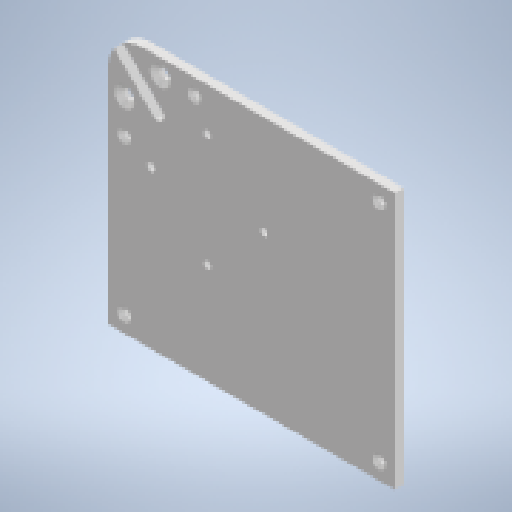
# Autodesk Inventor part: Mount plate UR
Saved by Autodesk Inventor 2024 (Build 280153000, 153)
## iProperties
Created: 2024-03-26
Part Number: Mount plate UR
Material: Generic
Document SubType Name: Modeling
Designer: jens1
Density: 1 g/cm^3
Appearance: Default
Author: jens1
Autodesk Inventor part; units mm, degrees
ref_plane "YZ Plane" through (0, 0, 0) normal (1, 0, 0) x (0, 1, 0)
ref_plane "XZ Plane" through (0, 0, 0) normal (0, 1, 0) x (-1, 0, 0)
ref_plane "XY Plane" through (0, 0, 0) normal (0, 0, 1) x (1, 0, 0)
sketch "Sketch1" plane through (0, 0, 0) normal (0, 0, 1) x (1, 0, 0)
  line L0 (0, 0) -> (335, 0)
  line L1 (335, 0) -> (335, 300)
  line L2 (335, 300) -> (0, 300)
  line L3 (0, 300) -> (0, 0)
  dimension "d0" = 335
  dimension "d1" = 300
  constraints: 8 end point, 2 parallel, 1 horizontal, 1 perpendicular
  measures "d0" distance of L2.end L1.end
  measures "d1" distance of L1.end L0.end
extrude "Plate" add sketch "Sketch1" along normal blind 10.5
sketch "Sketch3" plane through (0, 0, 10.5) normal (0, 0, 1) x (1, 0, 0)
  circle A0 centre (316.15, 18.85) radius 7.85
  line L0 (335, 0) -> (335, 300) projected
  line L1 (0, 0) -> (335, 0) projected
  circle A1 centre (316.15, 18.85) radius 4
  line L2 (0, 300) -> (0, 0) projected
  line L3 (335, 300) -> (0, 300) projected
  circle A2 centre (18.85, 199.55) radius 7.85
  circle A3 centre (100.45, 281.15) radius 7.85
  point P0 (18.85, 18.85)
  point P1 (316.15, 281.15)
  dimension "d4" = 15.7
  dimension "d5" = 18.85
  dimension "d6" = 18.85
  dimension "d7" = 8
  dimension "d8" = 18.85
  dimension "d9" = 18.85
  dimension "d10" = 18.85
  dimension "d11" = 18.85
  dimension "d19" = 18.85
  dimension "d20" = 18.85
  dimension "d21" = 15.7
  dimension "d22" = 15.7
  dimension "d23" = 180.7
  dimension "d24" = 215.7
  constraints: 4 centre point, 3 coincident
  measures "d4" diameter of A0
  measures "d5" distance from line of L0 A0.centre
  measures "d6" distance from line of L1 A0.centre
  measures "d7" diameter of A1
  measures "d8" distance from line of point (18.85, 18.85) L1
  measures "d9" distance from line of L2 point (18.85, 18.85)
  measures "d10" distance from line of L0 point (316.15, 281.15)
  measures "d11" distance from line of L3 point (316.15, 281.15)
  measures "d19" distance from line of L3 point (100.45, 281.15)
  measures "d20" distance from line of L2 point (18.85, 199.55)
  measures "d21" diameter of A3
  measures "d22" diameter of A2
  measures "d23" distance of point (18.85, 18.85) A2.centre
  measures "d24" distance of point (316.15, 281.15) point (100.45, 281.15)
hole "Small screw" at (18.85, 18.85, 10.5) at (316.15, 281.15, 10.5) at (316.15, 18.85, 10.5) at (18.85, 199.55, 10.5) at (100.45, 281.15, 10.5) direction (0, 0, -1) diameter 8 end through all countersink diameter 15.7 countersink angle 90
sketch "Sketch4" plane through (0, 0, 10.5) normal (0, 0, 1) x (1, 0, 0)
  circle A0 centre (100.45, 281.15) radius 7.85 projected
  circle A1 centre (18.85, 199.55) radius 7.85 projected
  circle A2 centre (18.85, 239.15) radius 11.75
  circle A3 centre (60.85, 281.15) radius 11.75
  circle A4 centre (18.85, 199.55) radius 4 projected
  circle A5 centre (18.85, 199.55) radius 7.85
  point P0 (0, 0)
  dimension "d25" = 23.5
  dimension "d26" = 23.5
  dimension "d27" = 0
  dimension "d28" = 0
  dimension "d29" = 39.6
  dimension "d30" = 15.7
  dimension "d31" = 39.6
  constraints: 3 centre point, 3 coincident
  measures "d25" diameter of A2
  measures "d26" diameter of A3
  measures "d27" vertical distance of A0.centre point (60.85, 281.15)
  measures "d28" horizontal distance of A1.centre point (18.85, 239.15)
  measures "d29" distance of point (18.85, 239.15) A1.centre
  measures "d30" diameter of A5
  measures "d31" distance of A0.centre A3.centre
hole "Big screw" at (60.85, 281.15, 10.5) at (18.85, 239.15, 10.5) direction (0, 0, -1) diameter 12 end through all countersink diameter 23.5 countersink angle 90
fillet "Stor runding" radius 40 1 edges at (0, 300, 5.25)
sketch "Sketch6" plane through (0, 0, 10.5) normal (0, 0, 1) x (1, 0, 0)
  arc A0 (40, 300) -> (0, 260) centre (40, 260) ccw projected
  line L0 (0, 260) -> (0, 0) projected
  line L1 (0, 0) -> (335, 0) projected
  line L2 (335, 0) -> (335, 300) projected
  line L3 (335, 300) -> (40, 300) projected
  circle A1 centre (18.85, 239.15) radius 11.75 projected
  circle A2 centre (60.85, 281.15) radius 11.75 projected
  circle A3 centre (100.45, 281.15) radius 7.85 projected
  circle A4 centre (18.85, 199.55) radius 7.85 projected
  circle A5 centre (316.15, 18.85) radius 7.85 projected
  circle A6 centre (316.15, 281.15) radius 7.85 projected
  circle A7 centre (18.85, 18.85) radius 7.85 projected
  line L4 (17.5207, 293.0859) -> (6.9141, 282.4793)
  line L5 (6.9141, 282.4793) -> (57.8257, 231.5676)
  line L6 (57.8257, 231.5676) -> (68.4324, 242.1743)
  line L7 (68.4324, 242.1743) -> (17.5207, 293.0859)
  arc A8 (40, 300) -> (0, 260) centre (40, 260) ccw projected
  dimension "d40" = 15
  dimension "d41" = 72
  dimension "d42" = 135
  constraints: 8 end point, 2 parallel, 2 point on circle, 1 perpendicular
  measures "d40" distance of L4.start L4.end
  measures "d41" distance of L5.end L4.end
  measures "d42" angle of L0 L4
extrude "Extrusion2" cut sketch "Sketch6" against normal up to next contours L4 A0 | L7 L6 L5 L4
fillet "Fillet2" radius 7.5 2 edges at (68.4324, 242.1743, 5.25) (57.8257, 231.5676, 5.25)
sketch "Sketch7" plane through (0, 0, 0) normal (0, 0, -1) x (-1, 0, 0)
  circle A0 centre (-116, 184) radius 74.5 projected
  circle A1 centre (-116, 250) radius 4.5 projected
  circle A2 centre (-182, 184) radius 4.5 projected
  circle A3 centre (-116, 118) radius 4.5 projected
  circle A4 centre (-116, 118) radius 4.5 projected
  circle A5 centre (-50, 184) radius 4.5 projected
  point P0 (0, 0)
extrude "Extrusion3" cut sketch "Sketch7" against normal up to next contours A1 | A2 | A3 | A5
equation "\"d5\" = d6"
equation "\"d8\" = d6"
equation "\"d9\" = d8"
equation "\"d10\" = d9"
equation "\"d11\" = d9"
equation "\"d19\" = d11"
equation "\"d20\" = d9"
equation "\"d21\" = d4"
equation "\"d22\" = d21"
equation "\"d31\" = d29"
body "Solid1"
